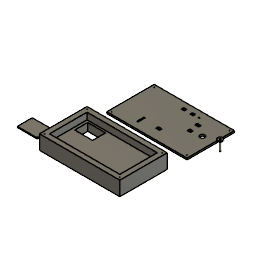
Smart Home system simulator case (Autodesk Fusion 360 design; units mm, degrees)
part number: 2026-07-06-12-17-13-399
Autodesk Fusion 360 part; units mm, degrees
sketch "Sketch1" plane through (0, 0, 0) normal (0, 1, 0) x (1, 0, 0)
  line L0 (-90, -62) -> (-90, 50)
  line L1 (-90, 50) -> (120, 50)
  line L2 (120, 50) -> (120, -62)
  line L3 (-90, -62) -> (120, -62)
  line L4 (-90, 50) -> (-105, 50)
  line L5 (-90, -62) -> (-105, -62)
  line L6 (135, 50) -> (120, 50)
  line L7 (135, -62) -> (120, -62)
  line L8 (120, -62) -> (120, -77)
  line L9 (120, 65) -> (120, 50)
  line L10 (-90, -62) -> (-90, -77)
  line L11 (-90, 65) -> (-90, 50)
  line L12 (-105, 65.7392) -> (135, 65.7392)
  line L13 (-105, -76.2608) -> (135, -76.2608)
  line L14 (135, 65.7392) -> (135, -76.2608)
  line L15 (-105, 65.7392) -> (-105, -76.2608)
  point P0 (-90, 50)
  point P1 (120, -62)
  dimension "d1" = 112
  dimension "d2" = 210
  dimension "d4" = 112
  dimension "d5" = 15
  dimension "d6" = 15
  dimension "d7" = 15
  dimension "d8" = 15
  dimension "d9" = 15
  dimension "d10" = 15
  dimension "d11" = 15
  dimension "d12" = 15
  dimension "d13" = 240
  dimension "d14" = 240
  constraint vertical L0
  constraint perpendicular L0 L1
  constraint perpendicular L1 L2
  constraint perpendicular L0 L4
  constraint perpendicular L3 L8
  constraint perpendicular L9 L12
  constraint perpendicular L13 L14
  constraint perpendicular L13 L15
  measures "d1" distance of P0 L0.start
  measures "d2" distance of P0 L1.end
  measures "d4" distance of L1.end P1
  measures "d5" distance of P0 L4.end
  measures "d6" distance of L0.start L5.end
  measures "d7" distance of L6.start L1.end
  measures "d8" distance of P1 L7.start
  measures "d9" distance of P1 L8.end
  measures "d10" distance of L9.start L1.end
  measures "d11" distance of L0.start L10.end
  measures "d12" distance of P0 L11.start
  measures "d13" distance of L12.start L12.end
  measures "d14" distance of L13.start L13.end
extrude "Extrude1" add sketch "Sketch1" along normal blind 3 contours L0 L1 L2 L3 makes body 1
sketch "Sketch2" plane through (0, 3, 0) normal (0, 1, 0) x (-1, 0, 0)
  line L0 (90, -50) -> (90, 62)
  line L1 (90, 62) -> (-120, 62)
  line L2 (-120, 62) -> (-120, -50)
  line L3 (-120, -50) -> (90, -50)
  line L4 (105, 77) -> (-135, 77)
  line L5 (-135, 77) -> (-135, -65)
  line L6 (-135, -65) -> (105, -65)
  line L7 (105, -65) -> (105, 77)
  dimension "d17" = 15
extrude "Extrude2" add sketch "Sketch2" along normal blind 20 separate body makes body 2
extrude "Extrude3" add 1 faces at (-20, 3, -12.6667) along direction (0, 1, 0) blind 10 on bodies 1 bodies 1 2
extrude "Extrude4" add 1 faces at (-20, 23, 72) along direction (0, 1, 0) blind 20 on bodies 1 bodies 1
sketch "Sketch3" plane through (0, 13, 0) normal (0, 1, 0) x (-1, 0, 0)
  line L0 (90, -50) -> (90, 62)
  line L1 (90, 62) -> (-120, 62)
  line L2 (-120, 62) -> (-120, -50)
  line L3 (-120, -50) -> (90, -50)
extrude "Extrude5" add 1 faces at (-20, 3, -60) along direction (0, -1, 0) blind 3 on bodies 1 bodies 1
extrude "Extrude6" add sketch "Sketch3" along normal blind 10 bodies 1
sketch "Sketch4" plane through (0, 23, 0) normal (0, 1, 0) x (-1, 0, 0)
  line L0 (-120, -50) -> (90, -50)
  line L1 (90, -50) -> (90, 62)
  line L2 (90, 62) -> (-120, 62)
  line L3 (-120, 62) -> (-120, -50)
  line L4 (82.25, -44.25) -> (82.25, -5.5)
  line L5 (82.25, -44.25) -> (28.75, -44.25)
  line L6 (82.25, -5.5) -> (28.75, -5.5)
  line L7 (28.75, -5.5) -> (28.75, -44.25)
  dimension "d30" = 38.75
  dimension "d31" = 53.5
  dimension "d32" = 53.5
  constraint perpendicular L0 L4
  constraint perpendicular L4 L5
  constraint perpendicular L4 L6
  measures "d30" distance of L4.start L4.end
  measures "d31" distance of L4.start L5.end
  measures "d32" distance of L4.end L6.end
extrude "Extrude7" cut sketch "Sketch4" against normal blind 40 contours L4 L5 L6 L7 bodies 1
sketch "Sketch5" plane through (0, 0, 0) normal (0, -1, 0) x (1, 0, 0)
  line L0 (-82.25, -5.5) -> (-28.75, -5.5)
  line L1 (-28.75, -5.5) -> (-28.75, -44.25)
  line L2 (-28.75, -44.25) -> (-82.25, -44.25)
  line L3 (-82.25, -44.25) -> (-82.25, -5.5)
  line L4 (-105, 77) -> (-105, -65)
  line L5 (-105, -65) -> (135, -65)
  line L6 (135, -65) -> (135, 77)
  line L7 (135, 77) -> (-105, 77)
  line L8 (-85.5537, -2.4963) -> (-24.2818, -2.4963)
  line L9 (-24.2818, -2.4963) -> (-24.2818, -47.202)
  line L10 (-24.2818, -47.202) -> (-85.5537, -47.202)
  line L11 (-85.5537, -47.202) -> (-85.5537, -2.4963)
  constraint horizontal L8
  constraint vertical L9
  constraint horizontal L10
  constraint vertical L11
extrude "Extrude8" add sketch "Sketch5" along normal blind 3 contours L8 L9 L10 L11 bodies 1
sketch "Sketch6" plane through (0, 0, 0) normal (0, 1, 0) x (1, 0, 0)
sketch "Sketch7" plane through (0, 0, 0) normal (0, 1, 0) x (1, 0, 0)
  line L0 (-137.7225, -51.0477) -> (-137.7225, -6.0477)
  line L1 (-137.7225, -51.0477) -> (-197.7225, -51.0477)
  line L2 (-137.7225, -6.0477) -> (-197.7225, -6.0477)
  line L3 (-197.7225, -51.0477) -> (-197.7225, -6.0477)
  dimension "d37" = 45
  dimension "d38" = 60
  dimension "d39" = 60
  constraint vertical L0
  constraint perpendicular L0 L1
  constraint perpendicular L0 L2
  measures "d37" distance of L0.start L0.end
  measures "d38" distance of L0.start L1.end
  measures "d39" distance of L0.end L2.end
extrude "Extrude9" add sketch "Sketch7" along normal blind 3 separate body makes body 3
sketch "Sketch8" plane through (0, -3, 0) normal (0, -1, 0) x (1, 0, 0)
  line L0 (-28.75, -44.25) -> (-82.25, -44.25)
  line L1 (-82.25, -44.25) -> (-82.25, -5.5)
  line L2 (-82.25, -5.5) -> (-28.75, -5.5)
  line L3 (-28.75, -5.5) -> (-28.75, -44.25)
  line L4 (-85.5537, -47.202) -> (-24.2818, -47.202)
  line L5 (-24.2818, -47.202) -> (-24.2818, -2.4963)
  line L6 (-24.2818, -2.4963) -> (-85.5537, -2.4963)
  line L7 (-85.5537, -2.4963) -> (-85.5537, -47.202)
extrude "Extrude10" cut sketch "Sketch8" against normal blind 2 bodies 1
extrude "Extrude11" cut 1 faces at (-25.7712, -1, -18.3994) along direction (0, 1, 0) blind 0.8 on bodies 1 bodies 1
extrude "Extrude12" cut 1 faces at (-25.7712, -0.2, -18.3994) along direction (0, 1, 0) blind 0.2 on bodies 1 bodies 1
sketch "Sketch11" plane through (0, 0, 0) normal (0, -1, 0) x (1, 0, 0)
  line L0 (-137.7225, 6.0477) -> (-137.7225, 51.0477)
  line L1 (-137.7225, 51.0477) -> (-197.7225, 51.0477)
  line L2 (-197.7225, 51.0477) -> (-197.7225, 6.0477)
  line L3 (-197.7225, 6.0477) -> (-137.7225, 6.0477)
  line L4 (-137.7225, 6.0477) -> (-139.3475, 6.0477)
  line L5 (-139.3475, 6.0477) -> (-139.3475, 7.6102)
  dimension "d84" = 1.625
  dimension "d85" = 1.5625
  constraint coincident L0.start L3.end
  constraint perpendicular L0 L4
  constraint perpendicular L4 L5
  measures "d84" distance of L0.start L4.end
  measures "d85" distance of L4.end L5.end
hole "Hole7" at (-139.3475, 0, 7.6102) direction (0, 1, 0) diameter 2.529 depth 3 tip angle 118 bodies 3
thread "Thread7" "ISO Metric profile 3.0 M3x0.5 M3x0.5 6H" thread offset 0 thread depth 7.4
sketch "Sketch12" plane through (0, 0, 0) normal (0, -1, 0) x (1, 0, 0)
  circle A0 centre (-139.3475, 7.6102) radius 1.2645
  line L0 (-137.7225, 6.0477) -> (-137.7225, 51.0477)
  line L1 (-137.7225, 51.0477) -> (-197.7225, 51.0477)
  line L2 (-197.7225, 51.0477) -> (-197.7225, 6.0477)
  line L3 (-197.7225, 6.0477) -> (-137.7225, 6.0477)
  line L4 (-197.7225, 6.0477) -> (-196.0975, 6.0477)
  line L5 (-196.0975, 6.0477) -> (-196.0975, 7.6102)
  dimension "d91" = 1.625
  dimension "d92" = 1.5625
  constraint coincident L2.end L3.start
  constraint perpendicular L2 L4
  constraint perpendicular L4 L5
  measures "d91" distance of L2.end L4.end
  measures "d92" distance of L4.end L5.end
hole "Hole8" at (-196.0975, 0, 7.6102) direction (0, 1, 0) diameter 2.529 depth 5 tip angle 118 bodies 3
thread "Thread8" "ISO Metric profile 3.0 M3x0.5 M3x0.5 6H" thread offset 0 thread depth 7.4
sketch "Sketch13" plane through (0, 0, 0) normal (0, -1, 0) x (1, 0, 0)
  circle A0 centre (-196.0975, 7.6102) radius 1.2645
  circle A1 centre (-139.3475, 7.6102) radius 1.2645
  line L0 (-137.7225, 6.0477) -> (-137.7225, 51.0477)
  line L1 (-137.7225, 51.0477) -> (-197.7225, 51.0477)
  line L2 (-197.7225, 51.0477) -> (-197.7225, 6.0477)
  line L3 (-197.7225, 6.0477) -> (-137.7225, 6.0477)
  line L4 (-137.7225, 51.0477) -> (-139.3475, 51.0477)
  line L5 (-139.3475, 51.0477) -> (-139.3475, 49.4852)
  dimension "d98" = 1.625
  dimension "d99" = 1.5625
  constraint coincident L0.end L1.start
  constraint perpendicular L0 L4
  constraint perpendicular L4 L5
  measures "d98" distance of L0.end L4.end
  measures "d99" distance of L4.end L5.end
hole "Hole9" at (-139.3475, 0, 49.4852) direction (0, 1, 0) diameter 2.529 depth 6 tip angle 118 bodies 3
thread "Thread9" "ISO Metric profile 3.0 M3x0.5 M3x0.5 6H" thread offset 0 thread depth 7.4
sketch "Sketch14" plane through (0, 0, 0) normal (0, -1, 0) x (1, 0, 0)
  circle A0 centre (-139.3475, 49.4852) radius 1.2645
  circle A1 centre (-196.0975, 7.6102) radius 1.2645
  circle A2 centre (-139.3475, 7.6102) radius 1.2645
  line L0 (-137.7225, 6.0477) -> (-137.7225, 51.0477)
  line L1 (-137.7225, 51.0477) -> (-197.7225, 51.0477)
  line L2 (-197.7225, 51.0477) -> (-197.7225, 6.0477)
  line L3 (-197.7225, 6.0477) -> (-137.7225, 6.0477)
  line L4 (-197.7225, 51.0477) -> (-196.0975, 51.0477)
  line L5 (-196.0975, 51.0477) -> (-196.0975, 49.4852)
  dimension "d105" = 1.625
  dimension "d106" = 1.5625
  constraint coincident L1.end L2.start
  constraint perpendicular L2 L4
  constraint perpendicular L4 L5
  measures "d105" distance of L1.end L4.end
  measures "d106" distance of L4.end L5.end
hole "Hole10" at (-196.0975, 0, 49.4852) direction (0, 1, 0) diameter 2.529 depth 4 tip angle 118 bodies 3
thread "Thread10" "ISO Metric profile 3.0 M3x0.5 M3x0.5 6H" thread offset 0 thread depth 7.4
sketch "Sketch15" plane through (0, 0, 0) normal (0, -1, 0) x (1, 0, 0)
  line L0 (-82.25, -5.5) -> (-28.75, -5.5)
  line L1 (-28.75, -5.5) -> (-28.75, -44.25)
  line L2 (-28.75, -44.25) -> (-82.25, -44.25)
  line L3 (-82.25, -44.25) -> (-82.25, -5.5)
  line L4 (-105, 77) -> (-105, -65)
  line L5 (-105, -65) -> (135, -65)
  line L6 (135, -65) -> (135, 77)
  line L7 (135, 77) -> (-105, 77)
  line L8 (-28.75, -44.25) -> (-27.125, -44.25)
  line L9 (-27.125, -44.25) -> (-27.125, -44.548)
  dimension "d112" = 1.625
  dimension "d113" = 0.298
  constraint coincident L1.end L2.start
  constraint perpendicular L1 L8
  constraint perpendicular L8 L9
  measures "d112" distance of L1.end L8.end
  measures "d113" distance of L8.end L9.end
hole "Hole11" at (-27.125, 0, -44.548) direction (0, 1, 0) diameter 2.529 depth 7 tip angle 118 bodies 1
thread "Thread11" "ISO Metric profile 3.0 M3x0.5 M3x0.5 6H" thread offset 0 thread depth 7.4
sketch "Sketch16" plane through (0, 0, 0) normal (0, -1, 0) x (1, 0, 0)
  circle A0 centre (-27.125, -44.548) radius 1.2645
  line L0 (-82.25, -5.5) -> (-28.75, -5.5)
  line L1 (-28.75, -5.5) -> (-28.75, -44.25)
  line L2 (-28.75, -44.25) -> (-82.25, -44.25)
  line L3 (-82.25, -44.25) -> (-82.25, -5.5)
  line L4 (-105, 77) -> (-105, -65)
  line L5 (-105, -65) -> (135, -65)
  line L6 (135, -65) -> (135, 77)
  line L7 (135, 77) -> (-105, 77)
  line L8 (-82.25, -44.25) -> (-83.875, -44.25)
  line L9 (-83.875, -44.25) -> (-83.875, -44.548)
  dimension "d119" = 1.625
  dimension "d120" = 0.298
  constraint coincident L2.end L3.start
  constraint perpendicular L3 L8
  constraint perpendicular L2 L9
  measures "d119" distance of L2.end L8.end
  measures "d120" distance of L8.end L9.end
hole "Hole12" at (-83.875, 0, -44.548) direction (0, 1, 0) diameter 2.529 depth 7 tip angle 118 bodies 1
thread "Thread12" "ISO Metric profile 3.0 M3x0.5 M3x0.5 6H" thread offset 0 thread depth 7.4
sketch "Sketch17" plane through (0, 0, 0) normal (0, -1, 0) x (1, 0, 0)
  circle A0 centre (-83.875, -44.548) radius 1.2645
  circle A1 centre (-27.125, -44.548) radius 1.2645
  line L0 (-82.25, -5.5) -> (-28.75, -5.5)
  line L1 (-28.75, -5.5) -> (-28.75, -44.25)
  line L2 (-28.75, -44.25) -> (-82.25, -44.25)
  line L3 (-82.25, -44.25) -> (-82.25, -5.5)
  line L4 (-105, 77) -> (-105, -65)
  line L5 (-105, -65) -> (135, -65)
  line L6 (135, -65) -> (135, 77)
  line L7 (135, 77) -> (-105, 77)
  line L8 (-28.75, -5.5) -> (-27.125, -5.5)
  line L9 (-27.125, -5.5) -> (-27.125, -5.202)
  dimension "d126" = 1.625
  dimension "d127" = 0.298
  constraint coincident L0.end L1.start
  constraint perpendicular L1 L8
  constraint perpendicular L8 L9
  measures "d126" distance of L0.end L8.end
  measures "d127" distance of L8.end L9.end
hole "Hole13" at (-27.125, 0, -5.202) direction (0, 1, 0) diameter 2.529 depth 7 tip angle 118 bodies 1
thread "Thread13" "ISO Metric profile 3.0 M3x0.5 M3x0.5 6H" thread offset 0 thread depth 7.4
sketch "Sketch18" plane through (0, 0, 0) normal (0, -1, 0) x (1, 0, 0)
  circle A0 centre (-27.125, -5.202) radius 1.2645
  circle A1 centre (-83.875, -44.548) radius 1.2645
  circle A2 centre (-27.125, -44.548) radius 1.2645
  line L0 (-82.25, -5.5) -> (-28.75, -5.5)
  line L1 (-28.75, -5.5) -> (-28.75, -44.25)
  line L2 (-28.75, -44.25) -> (-82.25, -44.25)
  line L3 (-82.25, -44.25) -> (-82.25, -5.5)
  line L4 (-105, 77) -> (-105, -65)
  line L5 (-105, -65) -> (135, -65)
  line L6 (135, -65) -> (135, 77)
  line L7 (135, 77) -> (-105, 77)
  line L8 (-82.25, -5.5) -> (-83.875, -5.5)
  line L9 (-83.875, -5.5) -> (-83.875, -5.202)
  dimension "d133" = 1.625
  dimension "d134" = 0.298
  constraint coincident L0.start L3.end
  constraint perpendicular L3 L8
  constraint perpendicular L8 L9
  measures "d133" distance of L0.start L8.end
  measures "d134" distance of L8.end L9.end
hole "Hole14" at (-83.875, 0, -5.202) direction (0, 1, 0) diameter 2.529 depth 7 tip angle 118 bodies 1
thread "Thread14" "ISO Metric profile 3.0 M3x0.5 M3x0.5 6H" thread offset 0 thread depth 7.4
sketch "Sketch19" plane through (0, 0, 0) normal (0, 1, 0) x (1, 0, 0)
  line L0 (-99.7579, 260.7276) -> (-99.7579, 118.7276)
  line L1 (-99.7579, 260.7276) -> (140.2421, 260.7276)
  line L2 (140.2421, 260.7276) -> (140.2421, 118.7276)
  line L3 (-99.7579, 118.7276) -> (140.2421, 118.7276)
  dimension "d140" = 142
  dimension "d141" = 240
  dimension "d142" = 142
  constraint vertical L0
  constraint perpendicular L0 L1
  constraint perpendicular L1 L2
  measures "d140" distance of L0.start L0.end
  measures "d141" distance of L0.start L1.end
  measures "d142" distance of L1.end L2.end
extrude "Extrude13" add sketch "Sketch19" along normal blind 5 separate body makes body 4
sketch "Sketch20" plane through (0, 5, 0) normal (0, 1, 0) x (-1, 0, 0)
  line L0 (99.7579, -260.7276) -> (99.7579, -118.7276)
  line L1 (99.7579, -118.7276) -> (-140.2421, -118.7276)
  line L2 (-140.2421, -118.7276) -> (-140.2421, -260.7276)
  line L3 (-140.2421, -260.7276) -> (99.7579, -260.7276)
  line L4 (99.7579, -260.7276) -> (92.2579, -260.7276)
  line L5 (92.2579, -260.7276) -> (92.2579, -253.2276)
  dimension "d145" = 7.5
  dimension "d146" = 7.5
  constraint coincident L0.start L3.end
  constraint perpendicular L0 L4
  constraint perpendicular L4 L5
  measures "d145" distance of L0.start L4.end
  measures "d146" distance of L4.end L5.end
hole "Hole15" at (-92.2579, 5, -253.2276) direction (0, -1, 0) diameter 2.529 depth 5 tip angle 118 bodies 4
thread "Thread15" "ISO Metric profile 3.0 M3x0.5 M3x0.5 6H" thread offset 0 thread depth 7.4
sketch "Sketch21" plane through (0, 5, 0) normal (0, 1, 0) x (-1, 0, 0)
  circle A0 centre (92.2579, -253.2276) radius 1.2645
  line L0 (99.7579, -260.7276) -> (99.7579, -118.7276)
  line L1 (99.7579, -118.7276) -> (-140.2421, -118.7276)
  line L2 (-140.2421, -118.7276) -> (-140.2421, -260.7276)
  line L3 (-140.2421, -260.7276) -> (99.7579, -260.7276)
  line L4 (-140.2421, -260.7276) -> (-132.7421, -260.7276)
  line L5 (-132.7421, -260.7276) -> (-132.7421, -253.2276)
  dimension "d152" = 7.5
  dimension "d153" = 7.5
  constraint coincident L2.end L3.start
  constraint perpendicular L2 L4
  constraint perpendicular L3 L5
  measures "d152" distance of L2.end L4.end
  measures "d153" distance of L4.end L5.end
hole "Hole16" at (132.7421, 5, -253.2276) direction (0, -1, 0) diameter 2.529 depth 5 tip angle 118 bodies 4
thread "Thread16" "ISO Metric profile 3.0 M3x0.5 M3x0.5 6H" thread offset 0 thread depth 7.4
sketch "Sketch22" plane through (0, 5, 0) normal (0, 1, 0) x (-1, 0, 0)
  circle A0 centre (-132.7421, -253.2276) radius 1.2645
  circle A1 centre (92.2579, -253.2276) radius 1.2645
  line L0 (99.7579, -260.7276) -> (99.7579, -118.7276)
  line L1 (99.7579, -118.7276) -> (-140.2421, -118.7276)
  line L2 (-140.2421, -118.7276) -> (-140.2421, -260.7276)
  line L3 (-140.2421, -260.7276) -> (99.7579, -260.7276)
  line L4 (99.7579, -118.7276) -> (92.2579, -118.7276)
  line L5 (92.2579, -118.7276) -> (92.2579, -126.2276)
  dimension "d159" = 7.5
  dimension "d160" = 7.5
  constraint coincident L0.end L1.start
  constraint perpendicular L0 L4
  constraint perpendicular L1 L5
  measures "d159" distance of L0.end L4.end
  measures "d160" distance of L4.end L5.end
hole "Hole17" at (-92.2579, 5, -126.2276) direction (0, -1, 0) diameter 2.529 depth 5 tip angle 118 bodies 4
thread "Thread17" "ISO Metric profile 3.0 M3x0.5 M3x0.5 6H" thread offset 0 thread depth 7.4
sketch "Sketch23" plane through (0, 5, 0) normal (0, 1, 0) x (-1, 0, 0)
  circle A0 centre (92.2579, -126.2276) radius 1.2645
  circle A1 centre (-132.7421, -253.2276) radius 1.2645
  circle A2 centre (92.2579, -253.2276) radius 1.2645
  line L0 (99.7579, -260.7276) -> (99.7579, -118.7276)
  line L1 (99.7579, -118.7276) -> (-140.2421, -118.7276)
  line L2 (-140.2421, -118.7276) -> (-140.2421, -260.7276)
  line L3 (-140.2421, -260.7276) -> (99.7579, -260.7276)
  line L4 (-140.2421, -118.7276) -> (-132.7421, -118.7276)
  line L5 (-132.7421, -118.7276) -> (-132.7421, -126.2276)
  dimension "d166" = 7.5
  dimension "d167" = 7.5
  constraint coincident L1.end L2.start
  constraint perpendicular L2 L4
  constraint perpendicular L1 L5
  measures "d166" distance of L1.end L4.end
  measures "d167" distance of L4.end L5.end
hole "Hole18" at (132.7421, 5, -126.2276) direction (0, -1, 0) diameter 2.529 depth 5 tip angle 118 bodies 4
thread "Thread18" "ISO Metric profile 3.0 M3x0.5 M3x0.5 6H" thread offset 0 thread depth 7.4
sketch "Sketch24" plane through (0, 43, 0) normal (0, 1, 0) x (-1, 0, 0)
  line L0 (90, -50) -> (-120, -50)
  line L1 (-120, -50) -> (-120, 62)
  line L2 (-120, 62) -> (90, 62)
  line L3 (90, 62) -> (90, -50)
  line L4 (105, -65) -> (105, 77)
  line L5 (105, 77) -> (-135, 77)
  line L6 (-135, 77) -> (-135, -65)
  line L7 (-135, -65) -> (105, -65)
  line L8 (105, -65) -> (97.5, -65)
  line L9 (97.5, -65) -> (97.5, -57.5)
  dimension "d173" = 7.5
  dimension "d174" = 7.5
  constraint coincident L4.start L7.end
  constraint perpendicular L4 L8
  constraint perpendicular L8 L9
  measures "d173" distance of L4.start L8.end
  measures "d174" distance of L8.end L9.end
hole "Hole19" at (-97.5, 43, -57.5) direction (0, -1, 0) diameter 2.529 depth 10 tip angle 118 bodies 1
thread "Thread19" "ISO Metric profile 3.0 M3x0.5 M3x0.5 6H" thread offset 0 thread depth 7.4
sketch "Sketch25" plane through (0, 43, 0) normal (0, 1, 0) x (-1, 0, 0)
  circle A0 centre (97.5, -57.5) radius 1.2645
  line L0 (90, -50) -> (-120, -50)
  line L1 (-120, -50) -> (-120, 62)
  line L2 (-120, 62) -> (90, 62)
  line L3 (90, 62) -> (90, -50)
  line L4 (105, -65) -> (105, 77)
  line L5 (105, 77) -> (-135, 77)
  line L6 (-135, 77) -> (-135, -65)
  line L7 (-135, -65) -> (105, -65)
  line L8 (-135, -65) -> (-127.5, -65)
  line L9 (-127.5, -65) -> (-127.5, -57.5)
  dimension "d180" = 7.5
  dimension "d181" = 7.5
  constraint coincident L6.end L7.start
  constraint perpendicular L6 L8
  constraint perpendicular L7 L9
  measures "d180" distance of L6.end L8.end
  measures "d181" distance of L8.end L9.end
hole "Hole20" at (127.5, 43, -57.5) direction (0, -1, 0) diameter 2.529 depth 10 tip angle 118 bodies 1
thread "Thread20" "ISO Metric profile 3.0 M3x0.5 M3x0.5 6H" thread offset 0 thread depth 7.4
sketch "Sketch26" plane through (0, 43, 0) normal (0, 1, 0) x (-1, 0, 0)
  circle A0 centre (-127.5, -57.5) radius 1.2645
  circle A1 centre (97.5, -57.5) radius 1.2645
  line L0 (90, -50) -> (-120, -50)
  line L1 (-120, -50) -> (-120, 62)
  line L2 (-120, 62) -> (90, 62)
  line L3 (90, 62) -> (90, -50)
  line L4 (105, -65) -> (105, 77)
  line L5 (105, 77) -> (-135, 77)
  line L6 (-135, 77) -> (-135, -65)
  line L7 (-135, -65) -> (105, -65)
  line L8 (-135, 77) -> (-127.5, 77)
  line L9 (-127.5, 77) -> (-127.5, 69.5)
  dimension "d187" = 7.5
  dimension "d188" = 7.5
  constraint coincident L5.end L6.start
  constraint perpendicular L6 L8
  constraint perpendicular L5 L9
  measures "d187" distance of L5.end L8.end
  measures "d188" distance of L8.end L9.end
hole "Hole21" at (127.5, 43, 69.5) direction (0, -1, 0) diameter 2.529 depth 10 tip angle 118 bodies 1
thread "Thread21" "ISO Metric profile 3.0 M3x0.5 M3x0.5 6H" thread offset 0 thread depth 7.4
sketch "Sketch27" plane through (0, 43, 0) normal (0, 1, 0) x (-1, 0, 0)
  circle A0 centre (-127.5, 69.5) radius 1.2645
  circle A1 centre (-127.5, -57.5) radius 1.2645
  circle A2 centre (97.5, -57.5) radius 1.2645
  line L0 (90, -50) -> (-120, -50)
  line L1 (-120, -50) -> (-120, 62)
  line L2 (-120, 62) -> (90, 62)
  line L3 (90, 62) -> (90, -50)
  line L4 (105, -65) -> (105, 77)
  line L5 (105, 77) -> (-135, 77)
  line L6 (-135, 77) -> (-135, -65)
  line L7 (-135, -65) -> (105, -65)
  line L8 (105, 77) -> (97.5, 77)
  line L9 (97.5, 77) -> (97.5, 69.5)
  dimension "d194" = 7.5
  dimension "d195" = 7.5
  constraint coincident L4.end L5.start
  constraint perpendicular L4 L8
  constraint perpendicular L5 L9
  measures "d194" distance of L4.end L8.end
  measures "d195" distance of L8.end L9.end
hole "Hole22" at (-97.5, 43, 69.5) direction (0, -1, 0) diameter 2.529 depth 10 tip angle 118 bodies 1
thread "Thread22" "ISO Metric profile 3.0 M3x0.5 M3x0.5 6H" thread offset 0 thread depth 7.4
sketch "Sketch28" plane through (0, 5, 0) normal (0, 1, 0) x (-1, 0, 0)
  circle A0 centre (-132.7421, -126.2276) radius 1.2645
  circle A1 centre (92.2579, -126.2276) radius 1.2645
  circle A2 centre (-132.7421, -253.2276) radius 1.2645
  circle A3 centre (92.2579, -253.2276) radius 1.2645
  line L0 (99.7579, -260.7276) -> (99.7579, -118.7276)
  line L1 (99.7579, -118.7276) -> (-140.2421, -118.7276)
  line L2 (-140.2421, -118.7276) -> (-140.2421, -260.7276)
  line L3 (-140.2421, -260.7276) -> (99.7579, -260.7276)
  line L4 (-140.2421, -260.7276) -> (-140.2421, -198.2276)
  line L5 (-140.2421, -198.2276) -> (-106.7421, -198.2276)
  dimension "d203" = 62.5
  dimension "d204" = 33.5
  constraint coincident L2.end L3.start
  constraint perpendicular L3 L4
  constraint perpendicular L2 L5
  measures "d203" distance of L2.end L4.end
  measures "d204" distance of L4.end L5.end
hole "Hole23" at (106.7421, 5, -198.2276) direction (0, -1, 0) diameter 14.5 depth 5 tip angle 180 bodies 4
sketch "Sketch29" plane through (0, 5, 0) normal (0, 1, 0) x (-1, 0, 0)
  circle A0 centre (-106.7421, -198.2276) radius 7.25
  circle A1 centre (-132.7421, -126.2276) radius 1.2645
  circle A2 centre (92.2579, -126.2276) radius 1.2645
  circle A3 centre (-132.7421, -253.2276) radius 1.2645
  circle A4 centre (92.2579, -253.2276) radius 1.2645
  line L0 (99.7579, -260.7276) -> (99.7579, -118.7276)
  line L1 (99.7579, -118.7276) -> (-140.2421, -118.7276)
  line L2 (-140.2421, -118.7276) -> (-140.2421, -260.7276)
  line L3 (-140.2421, -260.7276) -> (99.7579, -260.7276)
  line L4 (-4.9421, -244.1526) -> (-13.5421, -244.1526)
  line L5 (-13.5421, -244.1526) -> (-13.5421, -237.3026)
  line L6 (-13.5421, -237.3026) -> (-4.9421, -237.3026)
  line L7 (-4.9421, -244.1526) -> (-4.9421, -237.3026)
  dimension "d210" = 8.6
  dimension "d211" = 6.85
  dimension "d212" = 8.6
  constraint perpendicular L4 L5
  constraint perpendicular L5 L6
  measures "d210" distance of L4.start L4.end
  measures "d211" distance of L4.end L5.end
  measures "d212" distance of L5.end L6.end
extrude "Extrude14" cut sketch "Sketch29" against normal blind 10 contours L4 L5 L6 L7 bodies 4
sketch "Sketch30" plane through (0, 5, 0) normal (0, 1, 0) x (-1, 0, 0)
  line L0 (-4.9421, -237.3026) -> (-4.9421, -244.1526)
  line L1 (-4.9421, -244.1526) -> (-13.5421, -244.1526)
  line L2 (-13.5421, -244.1526) -> (-13.5421, -237.3026)
  line L3 (-13.5421, -237.3026) -> (-4.9421, -237.3026)
  circle A0 centre (-106.7421, -198.2276) radius 7.25
  circle A1 centre (-132.7421, -126.2276) radius 1.2645
  circle A2 centre (92.2579, -126.2276) radius 1.2645
  circle A3 centre (-132.7421, -253.2276) radius 1.2645
  circle A4 centre (92.2579, -253.2276) radius 1.2645
  line L4 (99.7579, -260.7276) -> (99.7579, -118.7276)
  line L5 (99.7579, -118.7276) -> (-140.2421, -118.7276)
  line L6 (-140.2421, -118.7276) -> (-140.2421, -260.7276)
  line L7 (-140.2421, -260.7276) -> (99.7579, -260.7276)
  line L8 (-30.9921, -244.2776) -> (-39.5921, -244.2776)
  line L9 (-39.5921, -244.2776) -> (-39.5921, -237.4276)
  line L10 (-30.9921, -244.2776) -> (-30.9921, -237.4276)
  line L11 (-30.9921, -237.4276) -> (-39.5921, -237.4276)
  dimension "d217" = 8.6
  dimension "d218" = 6.85
  dimension "d219" = 6.85
  constraint perpendicular L8 L9
  constraint perpendicular L8 L10
  measures "d217" distance of L8.start L8.end
  measures "d218" distance of L8.end L9.end
  measures "d219" distance of L8.start L10.end
extrude "Extrude15" cut sketch "Sketch30" against normal blind 15 contours L8 L9 L10 L11 bodies 4
sketch "Sketch31" plane through (0, 5, 0) normal (0, 1, 0) x (-1, 0, 0)
  line L0 (-39.5921, -237.4276) -> (-30.9921, -237.4276)
  line L1 (-30.9921, -237.4276) -> (-30.9921, -244.2776)
  line L2 (-30.9921, -244.2776) -> (-39.5921, -244.2776)
  line L3 (-39.5921, -244.2776) -> (-39.5921, -237.4276)
  line L4 (-4.9421, -237.3026) -> (-4.9421, -244.1526)
  line L5 (-4.9421, -244.1526) -> (-13.5421, -244.1526)
  line L6 (-13.5421, -244.1526) -> (-13.5421, -237.3026)
  line L7 (-13.5421, -237.3026) -> (-4.9421, -237.3026)
  circle A0 centre (-106.7421, -198.2276) radius 7.25
  circle A1 centre (-132.7421, -126.2276) radius 1.2645
  circle A2 centre (92.2579, -126.2276) radius 1.2645
  circle A3 centre (-132.7421, -253.2276) radius 1.2645
  circle A4 centre (92.2579, -253.2276) radius 1.2645
  line L8 (99.7579, -260.7276) -> (99.7579, -118.7276)
  line L9 (99.7579, -118.7276) -> (-140.2421, -118.7276)
  line L10 (-140.2421, -118.7276) -> (-140.2421, -260.7276)
  line L11 (-140.2421, -260.7276) -> (99.7579, -260.7276)
  line L12 (-51.9941, -242.1776) -> (-55.3541, -242.1776)
  line L13 (-51.9941, -242.1776) -> (-51.9941, -240.2676)
  line L14 (-51.9941, -240.2676) -> (-55.3541, -240.2676)
  line L15 (-55.3541, -242.1776) -> (-55.3541, -240.2676)
  dimension "d226" = 3.36
  dimension "d227" = 1.91
  dimension "d228" = 3.36
  constraint perpendicular L12 L13
  constraint perpendicular L13 L14
  measures "d226" distance of L12.start L12.end
  measures "d227" distance of L12.start L13.end
  measures "d228" distance of L13.end L14.end
extrude "Extrude16" cut sketch "Sketch31" against normal blind 8 contours L12 L13 L14 L15 bodies 4
sketch "Sketch32" plane through (0, 5, 0) normal (0, 1, 0) x (-1, 0, 0)
  line L0 (99.7579, -260.7276) -> (99.7579, -118.7276)
  line L1 (99.7579, -118.7276) -> (-140.2421, -118.7276)
  line L2 (-140.2421, -118.7276) -> (-140.2421, -260.7276)
  line L3 (-140.2421, -260.7276) -> (99.7579, -260.7276)
  circle A0 centre (92.2579, -253.2276) radius 1.2645
  circle A1 centre (-132.7421, -253.2276) radius 1.2645
  circle A2 centre (92.2579, -126.2276) radius 1.2645
  circle A3 centre (-132.7421, -126.2276) radius 1.2645
  circle A4 centre (-106.7421, -198.2276) radius 7.25
  line L4 (-4.9421, -237.3026) -> (-4.9421, -244.1526)
  line L5 (-4.9421, -244.1526) -> (-13.5421, -244.1526)
  line L6 (-13.5421, -244.1526) -> (-13.5421, -237.3026)
  line L7 (-13.5421, -237.3026) -> (-4.9421, -237.3026)
  line L8 (-39.5921, -237.4276) -> (-30.9921, -237.4276)
  line L9 (-30.9921, -237.4276) -> (-30.9921, -244.2776)
  line L10 (-30.9921, -244.2776) -> (-39.5921, -244.2776)
  line L11 (-39.5921, -244.2776) -> (-39.5921, -237.4276)
  line L12 (-55.3541, -240.2676) -> (-51.9941, -240.2676)
  line L13 (-51.9941, -240.2676) -> (-51.9941, -242.1776)
  line L14 (-51.9941, -242.1776) -> (-55.3541, -242.1776)
  line L15 (-55.3541, -242.1776) -> (-55.3541, -240.2676)
  line L16 (30.0279, -139.2576) -> (26.4879, -139.2576)
  line L17 (26.4879, -139.2576) -> (26.4879, -160.5776)
  line L18 (30.0279, -139.2576) -> (30.0279, -160.5776)
  line L19 (30.0279, -160.5776) -> (26.4879, -160.5776)
  dimension "d233" = 3.54
  dimension "d234" = 21.32
  dimension "d235" = 21.32
  constraint perpendicular L16 L17
  constraint perpendicular L16 L18
  measures "d233" distance of L16.start L16.end
  measures "d234" distance of L16.end L17.end
  measures "d235" distance of L16.start L18.end
extrude "Extrude17" cut sketch "Sketch32" against normal blind 50 contours L16 L17 L18 L19 bodies 4
sketch "Sketch33" plane through (0, 5, 0) normal (0, 1, 0) x (-1, 0, 0)
  line L0 (-55.3541, -240.2676) -> (-51.9941, -240.2676)
  line L1 (-51.9941, -240.2676) -> (-51.9941, -242.1776)
  line L2 (-51.9941, -242.1776) -> (-55.3541, -242.1776)
  line L3 (-55.3541, -242.1776) -> (-55.3541, -240.2676)
  line L4 (-39.5921, -237.4276) -> (-30.9921, -237.4276)
  line L5 (-30.9921, -237.4276) -> (-30.9921, -244.2776)
  line L6 (-30.9921, -244.2776) -> (-39.5921, -244.2776)
  line L7 (-39.5921, -244.2776) -> (-39.5921, -237.4276)
  line L8 (-4.9421, -237.3026) -> (-4.9421, -244.1526)
  line L9 (-4.9421, -244.1526) -> (-13.5421, -244.1526)
  line L10 (-13.5421, -244.1526) -> (-13.5421, -237.3026)
  line L11 (-13.5421, -237.3026) -> (-4.9421, -237.3026)
  circle A0 centre (-106.7421, -198.2276) radius 7.25
  circle A1 centre (-132.7421, -126.2276) radius 1.2645
  circle A2 centre (92.2579, -126.2276) radius 1.2645
  circle A3 centre (-132.7421, -253.2276) radius 1.2645
  circle A4 centre (92.2579, -253.2276) radius 1.2645
  line L12 (99.7579, -260.7276) -> (99.7579, -118.7276)
  line L13 (99.7579, -118.7276) -> (-140.2421, -118.7276)
  line L14 (-140.2421, -118.7276) -> (-140.2421, -260.7276)
  line L15 (-140.2421, -260.7276) -> (99.7579, -260.7276)
  line L16 (26.4879, -160.5776) -> (26.4879, -139.2576)
  line L17 (26.4879, -139.2576) -> (30.0279, -139.2576)
  line L18 (30.0279, -139.2576) -> (30.0279, -160.5776)
  line L19 (30.0279, -160.5776) -> (26.4879, -160.5776)
  line L20 (-78.9921, -197.9776) -> (-69.4921, -197.9776)
  line L21 (-78.9921, -197.9776) -> (-78.9921, -190.4776)
  line L22 (-69.4921, -197.9776) -> (-69.4921, -190.4776)
  line L23 (-69.4921, -190.4776) -> (-78.9921, -190.4776)
  dimension "d240" = 9.5
  dimension "d241" = 7.5
  dimension "d242" = 7.5
  constraint perpendicular L20 L21
  constraint perpendicular L20 L22
  measures "d240" distance of L20.start L20.end
  measures "d241" distance of L20.start L21.end
  measures "d242" distance of L20.end L22.end
extrude "Extrude18" cut sketch "Sketch33" against normal blind 35 contours L20 L21 L22 L23 bodies 4
sketch "Sketch34" plane through (0, 5, 0) normal (0, 1, 0) x (-1, 0, 0)
  line L0 (26.4879, -160.5776) -> (26.4879, -139.2576)
  line L1 (26.4879, -139.2576) -> (30.0279, -139.2576)
  line L2 (30.0279, -139.2576) -> (30.0279, -160.5776)
  line L3 (30.0279, -160.5776) -> (26.4879, -160.5776)
  line L4 (99.7579, -260.7276) -> (99.7579, -118.7276)
  line L5 (99.7579, -118.7276) -> (-140.2421, -118.7276)
  line L6 (-140.2421, -118.7276) -> (-140.2421, -260.7276)
  line L7 (-140.2421, -260.7276) -> (99.7579, -260.7276)
  circle A0 centre (92.2579, -253.2276) radius 1.2645
  circle A1 centre (-132.7421, -253.2276) radius 1.2645
  circle A2 centre (92.2579, -126.2276) radius 1.2645
  circle A3 centre (-132.7421, -126.2276) radius 1.2645
  circle A4 centre (-106.7421, -198.2276) radius 7.25
  line L8 (-4.9421, -237.3026) -> (-4.9421, -244.1526)
  line L9 (-4.9421, -244.1526) -> (-13.5421, -244.1526)
  line L10 (-13.5421, -244.1526) -> (-13.5421, -237.3026)
  line L11 (-13.5421, -237.3026) -> (-4.9421, -237.3026)
  line L12 (-39.5921, -237.4276) -> (-30.9921, -237.4276)
  line L13 (-30.9921, -237.4276) -> (-30.9921, -244.2776)
  line L14 (-30.9921, -244.2776) -> (-39.5921, -244.2776)
  line L15 (-39.5921, -244.2776) -> (-39.5921, -237.4276)
  line L16 (-55.3541, -240.2676) -> (-51.9941, -240.2676)
  line L17 (-51.9941, -240.2676) -> (-51.9941, -242.1776)
  line L18 (-51.9941, -242.1776) -> (-55.3541, -242.1776)
  line L19 (-55.3541, -242.1776) -> (-55.3541, -240.2676)
  line L20 (-69.4921, -190.4776) -> (-69.4921, -197.9776)
  line L21 (-69.4921, -197.9776) -> (-78.9921, -197.9776)
  line L22 (-78.9921, -197.9776) -> (-78.9921, -190.4776)
  line L23 (-78.9921, -190.4776) -> (-69.4921, -190.4776)
  circle A5 centre (-171.5603, -186.5537) radius 2.5
  dimension "d245" = 5
  measures "d245" diameter of A5
extrude "Extrude19" add sketch "Sketch34" along normal blind 28 separate body contours A5 makes body 5
sketch "Sketch35" plane through (0, 33, 0) normal (0, 1, 0) x (-1, 0, 0)
  circle A0 centre (-171.5603, -186.5537) radius 2.5
  circle A1 centre (-171.5603, -186.5537) radius 7.5
  dimension "d248" = 15
  constraint concentric A0 A1
  measures "d248" diameter of A1
extrude "Extrude20" add sketch "Sketch35" along normal blind 3 separate body makes body 6
sketch "Sketch36" plane through (0, 5, 0) normal (0, 1, 0) x (-1, 0, 0)
  line L0 (26.4879, -160.5776) -> (26.4879, -139.2576)
  line L1 (26.4879, -139.2576) -> (30.0279, -139.2576)
  line L2 (30.0279, -139.2576) -> (30.0279, -160.5776)
  line L3 (30.0279, -160.5776) -> (26.4879, -160.5776)
  line L4 (99.7579, -260.7276) -> (99.7579, -118.7276)
  line L5 (99.7579, -118.7276) -> (-140.2421, -118.7276)
  line L6 (-140.2421, -118.7276) -> (-140.2421, -260.7276)
  line L7 (-140.2421, -260.7276) -> (99.7579, -260.7276)
  circle A0 centre (92.2579, -253.2276) radius 1.2645
  circle A1 centre (-132.7421, -253.2276) radius 1.2645
  circle A2 centre (92.2579, -126.2276) radius 1.2645
  circle A3 centre (-132.7421, -126.2276) radius 1.2645
  circle A4 centre (-106.7421, -198.2276) radius 7.25
  line L8 (-4.9421, -237.3026) -> (-4.9421, -244.1526)
  line L9 (-4.9421, -244.1526) -> (-13.5421, -244.1526)
  line L10 (-13.5421, -244.1526) -> (-13.5421, -237.3026)
  line L11 (-13.5421, -237.3026) -> (-4.9421, -237.3026)
  line L12 (-39.5921, -237.4276) -> (-30.9921, -237.4276)
  line L13 (-30.9921, -237.4276) -> (-30.9921, -244.2776)
  line L14 (-30.9921, -244.2776) -> (-39.5921, -244.2776)
  line L15 (-39.5921, -244.2776) -> (-39.5921, -237.4276)
  line L16 (-55.3541, -240.2676) -> (-51.9941, -240.2676)
  line L17 (-51.9941, -240.2676) -> (-51.9941, -242.1776)
  line L18 (-51.9941, -242.1776) -> (-55.3541, -242.1776)
  line L19 (-55.3541, -242.1776) -> (-55.3541, -240.2676)
  line L20 (-69.4921, -190.4776) -> (-69.4921, -197.9776)
  line L21 (-69.4921, -197.9776) -> (-78.9921, -197.9776)
  line L22 (-78.9921, -197.9776) -> (-78.9921, -190.4776)
  line L23 (-78.9921, -190.4776) -> (-69.4921, -190.4776)
  line L24 (-76.9721, -223.9276) -> (-65.8721, -223.9276)
  line L25 (-65.8721, -223.9276) -> (-65.8721, -216.9276)
  line L26 (-76.9721, -223.9276) -> (-76.9721, -216.9276)
  line L27 (-65.8721, -216.9276) -> (-76.9721, -216.9276)
  dimension "d253" = 11.1
  dimension "d254" = 7
  dimension "d255" = 7
  constraint perpendicular L24 L25
  constraint perpendicular L24 L26
  measures "d253" distance of L24.start L24.end
  measures "d254" distance of L24.end L25.end
  measures "d255" distance of L24.start L26.end
extrude "Extrude21" cut sketch "Sketch36" against normal blind 60 contours L24 L25 L26 L27 bodies 4
sketch "Sketch37" plane through (0, 5, 0) normal (0, 1, 0) x (-1, 0, 0)
  line L0 (-69.4921, -190.4776) -> (-69.4921, -197.9776)
  line L1 (-69.4921, -197.9776) -> (-78.9921, -197.9776)
  line L2 (-78.9921, -197.9776) -> (-78.9921, -190.4776)
  line L3 (-78.9921, -190.4776) -> (-69.4921, -190.4776)
  line L4 (-55.3541, -240.2676) -> (-51.9941, -240.2676)
  line L5 (-51.9941, -240.2676) -> (-51.9941, -242.1776)
  line L6 (-51.9941, -242.1776) -> (-55.3541, -242.1776)
  line L7 (-55.3541, -242.1776) -> (-55.3541, -240.2676)
  line L8 (-39.5921, -237.4276) -> (-30.9921, -237.4276)
  line L9 (-30.9921, -237.4276) -> (-30.9921, -244.2776)
  line L10 (-30.9921, -244.2776) -> (-39.5921, -244.2776)
  line L11 (-39.5921, -244.2776) -> (-39.5921, -237.4276)
  line L12 (-4.9421, -237.3026) -> (-4.9421, -244.1526)
  line L13 (-4.9421, -244.1526) -> (-13.5421, -244.1526)
  line L14 (-13.5421, -244.1526) -> (-13.5421, -237.3026)
  line L15 (-13.5421, -237.3026) -> (-4.9421, -237.3026)
  circle A0 centre (-106.7421, -198.2276) radius 7.25
  circle A1 centre (-132.7421, -126.2276) radius 1.2645
  circle A2 centre (92.2579, -126.2276) radius 1.2645
  circle A3 centre (-132.7421, -253.2276) radius 1.2645
  circle A4 centre (92.2579, -253.2276) radius 1.2645
  line L16 (99.7579, -260.7276) -> (99.7579, -118.7276)
  line L17 (99.7579, -118.7276) -> (-140.2421, -118.7276)
  line L18 (-140.2421, -118.7276) -> (-140.2421, -260.7276)
  line L19 (-140.2421, -260.7276) -> (99.7579, -260.7276)
  line L20 (26.4879, -160.5776) -> (26.4879, -139.2576)
  line L21 (26.4879, -139.2576) -> (30.0279, -139.2576)
  line L22 (30.0279, -139.2576) -> (30.0279, -160.5776)
  line L23 (30.0279, -160.5776) -> (26.4879, -160.5776)
  line L24 (-65.8721, -216.9276) -> (-65.8721, -223.9276)
  line L25 (-65.8721, -223.9276) -> (-76.9721, -223.9276)
  line L26 (-76.9721, -223.9276) -> (-76.9721, -216.9276)
  line L27 (-76.9721, -216.9276) -> (-65.8721, -216.9276)
  line L28 (-16.1921, -149.7276) -> (-16.1921, -156.7276)
  line L29 (-16.1921, -156.7276) -> (-27.2921, -156.7276)
  line L30 (-16.1921, -149.7276) -> (-27.2921, -149.7276)
  line L31 (-27.2921, -156.7276) -> (-27.2921, -149.7276)
  dimension "d260" = 7
  dimension "d261" = 11.1
  dimension "d262" = 11.1
  constraint perpendicular L28 L29
  constraint perpendicular L28 L30
  measures "d260" distance of L28.start L28.end
  measures "d261" distance of L28.end L29.end
  measures "d262" distance of L28.start L30.end
extrude "Extrude22" cut sketch "Sketch37" against normal blind 20 contours L28 L29 L30 L31 bodies 4
